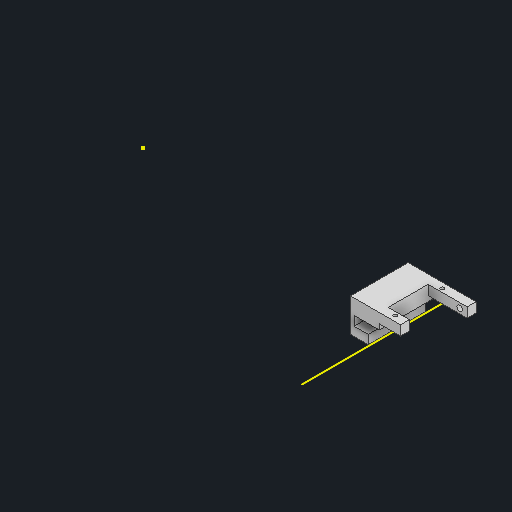
# Autodesk Inventor part: obj_3_外壳.STL
Saved by Autodesk Inventor 2025 (Build 290162000, 162)
## iProperties
Created: 2026-04-25
Part Number: obj_3_外壳.STL
Material: 常规
Document SubType Name: Modeling
Designer: XH
Density: 1 g/cm^3
Appearance: 默认
Author: XH
Autodesk Inventor part; units mm, degrees
ref_plane "YZ Plane" through (0, 0, 0) normal (1, 0, 0) x (0, 1, 0)
ref_plane "XZ Plane" through (0, 0, 0) normal (0, 1, 0) x (-1, 0, 0)
ref_plane "XY Plane" through (0, 0, 0) normal (0, 0, 1) x (1, 0, 0)
sketch "草图2" plane through (0, 0, 0) normal (0, 0, 1) x (1, 0, 0)
  line L0 (149.1878, 129.8039) -> (177.4063, 129.8039) projected
  line L1 (177.4063, 129.8039) -> (177.4063, 124.3039) projected
  line L2 (177.4063, 124.3039) -> (165.4062, 124.3039) projected
  line L3 (165.4062, 124.3039) -> (165.4062, 121.3039) projected
  line L4 (165.4062, 121.3039) -> (151.1878, 121.3039) projected
  line L5 (151.1878, 116.0039) -> (159.1878, 116.0039) projected
  line L6 (151.1878, 121.3039) -> (151.1878, 116.0039) projected
  line L7 (159.1878, 116.0039) -> (159.1878, 114.0039) projected
  line L8 (159.1878, 114.0039) -> (149.1878, 114.0039) projected
  line L9 (149.1878, 114.0039) -> (149.1878, 129.8039) projected
  point P0 (0, 0)
extrude "拉伸1" add sketch "草图2" along normal blind 32.5
sketch "草图3" plane through (165.4062, 124.3039, 0) normal (0, -1, 0) x (1, 0, 0)
  line L0 (0, 0) -> (0, 32.5) projected
  line L1 (12, 0) -> (12, 32.5) projected
  line L2 (0, 27.4986) -> (12, 27.4986)
  line L3 (12, 27.4986) -> (12, 4.9993)
  line L4 (12, 4.9993) -> (0, 4.9993)
  line L5 (0, 4.9993) -> (0, 27.4986)
  point P0 (-165.4062, 0)
  constraints: 8 end point, 2 parallel, 2 point on line, 1 horizontal, 1 perpendicular
extrude "拉伸2" cut sketch "草图3" against normal blind 24.5
sketch "草图4" plane through (165.4062, 124.3039, 32.5) normal (0, -1, 0) x (1, 0, 0)
  circle A0 centre (5.9961, -3.0044) radius 1
  point P0 (-165.4062, -32.5)
  dimension "d4" = 2
  constraints: 1 centre point
  measures "d4" diameter of A0
extrude "拉伸3" cut sketch "草图4" against normal blind 24.5
ref_plane "工作平面1" through (0, 0, 16.25) normal (0, 0, 1) x (1, 0, 0)
mirror "镜像1" about plane through (0, 0, 16.25) normal (0, 0, 1) of "拉伸3"
move faces "移动2" translate (0, -3, 0) faces at (152.5211, 114.0039, 10.8333)
sketch "草图5" plane through (149.1878, 111.0039, 0) normal (0, -1, 0) x (1, 0, 0)
  line L0 (10.75, -10.0255) -> (10.75, 70.5469) projected
  point P0 (-149.1878, 0)
sketch "草图6" plane through (0, 0, 0) normal (0, 0, -1) x (-1, 0, 0)
  circle A0 centre (-153.0103, 125.7656) radius 1.5
  circle A1 centre (-161.6582, 125.7656) radius 1.5
  point P0 (0, 0)
  dimension "d13" = 3
  dimension "d14" = 3
  constraints: 2 centre point
  measures "d13" diameter of A0
  measures "d14" diameter of A1
extrude "拉伸4" cut sketch "草图6" against normal blind 10
move faces "移动3" translate (10, 0, 0) faces at (177.4063, 127.9705, 3.3329)
sketch "草图7" plane through (0, 0, 0) normal (0, 0, -1) x (-1, 0, 0)
  circle A0 centre (-183.123, 127.0539) radius 1.5
  line L0 (-187.4063, 129.8039) -> (-187.4063, 124.3039) projected
  line L1 (-187.4063, 127.0539) -> (-179.6204, 127.0539)
  point P0 (0, 0)
  dimension "d20" = 3
  constraints: 2 end point, 1 centre point, 1 horizontal, 1 midpoint, 1 point on line
  measures "d20" diameter of A0
extrude "拉伸5" cut sketch "草图7" against normal blind 10
